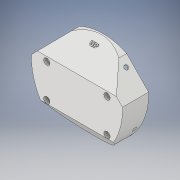
# Autodesk Inventor part: DGB Cover 2
Saved by Autodesk Inventor 2018 (Build 220112000, 112)
## iProperties
Created: 2019-02-18
Part Number: DGB Cover 2
Material: ABS Plastic
Document SubType Name: Modeling
Designer: Joe
Density: 1.06 g/cm^3
Appearance: Smooth - White
Author: Joe
Autodesk Inventor part; units mm, degrees
(part 1 of 16)
ref_plane "YZ Plane" through (0, 0, 0) normal (1, 0, 0) x (0, 1, 0)
ref_plane "Work Plane1" through (0, 0, 0) normal (0, 0, 1) x (1, 0, 0)
sketch "Sketch1" plane through (0, 0, 0) normal (0, 0, 1) x (1, 0, 0)
  arc A0 (-69.2264, 99.4238) -> (-77.754, 69.3573) centre (-45.7832, 76.5321) ccw
  line L0 (-61.6428, -2.4333) -> (-77.754, 69.3573)
  arc A1 (-61.6428, -2.4333) -> (-56.4257, -9.5833) centre (-50.8, 0) ccw
  line L1 (-56.4257, -9.5833) -> (-18.6452, -31.7617)
  arc A2 (-18.6452, -31.7617) -> (18.6452, -31.7617) centre (0, 0) ccw
  line L2 (56.4257, -9.5833) -> (18.6452, -31.7617)
  arc A3 (56.4257, -9.5833) -> (61.6428, -2.4333) centre (50.8, 0) ccw
  line L3 (77.754, 69.3573) -> (61.6428, -2.4333)
  arc A4 (77.754, 69.3573) -> (69.2264, 99.4238) centre (45.7832, 76.5321) ccw
  line L4 (69.2264, 99.4238) -> (23.4432, 146.3102)
  arc A5 (23.4432, 146.3102) -> (-23.4432, 146.3102) centre (0, 123.4186) ccw
  line L5 (-23.4432, 146.3102) -> (-69.2264, 99.4238)
  circle A6 centre (45.7832, 76.5321) radius 9.5631
  circle A7 centre (0, 123.4186) radius 9.5631
  circle A8 centre (63.5, 38.1) radius 2.4892
  circle A9 centre (0, 0) radius 14.2951
  circle A10 centre (0, 41.9862) radius 14.2951
  circle A11 centre (-63.5, 38.1) radius 2.4892
  circle A12 centre (50.8, 0) radius 2.4892
  circle A13 centre (-45.7832, 76.5321) radius 9.5631
  circle A14 centre (-50.8, 0) radius 2.4892
  arc A15 (60.8674, 81.4802) -> (51.089, 91.4942) centre (45.7832, 76.5321) ccw
  arc A16 (48.9582, 94.5106) -> (51.089, 91.4942) centre (52.1586, 94.5106) ccw
  line L6 (48.9582, 94.5106) -> (48.9582, 95.9294)
  arc A17 (49.8285, 98.1233) -> (48.9582, 95.9294) centre (52.1586, 95.9294) ccw
  arc A18 (49.8285, 98.1233) -> (51.2978, 101.2528) centre (45.7832, 101.9321) ccw
  arc A19 (56.764, 103.0974) -> (51.2978, 101.2528) centre (54.4742, 100.8615) ccw
  line L7 (56.764, 103.0974) -> (64.6832, 94.9874)
  arc A20 (71.3491, 83.1797) -> (64.6832, 94.9874) centre (45.7832, 76.5321) ccw
  arc A21 (68.1755, 79.1748) -> (71.3491, 83.1797) centre (68.2517, 82.3743) ccw
  line L8 (63.8322, 79.2782) -> (68.1755, 79.1748)
  arc A22 (60.8674, 81.4802) -> (63.8322, 79.2782) centre (63.9084, 82.4777) ccw
  arc A23 (42.8406, 46.4191) -> (46.4544, 45.6166) centre (45.7832, 51.1321) ccw
  arc A24 (48.7374, 45.0177) -> (46.4544, 45.6166) centre (46.841, 42.4396) ccw
  line L9 (56.7832, 39.0993) -> (48.7374, 45.0177)
  arc A25 (58.0348, 37.0983) -> (56.7832, 39.0993) centre (54.8868, 36.5212) ccw
  arc A26 (58.0348, 37.0983) -> (60.7938, 33.2473) centre (63.5, 38.1) ccw
  arc A27 (62.3577, 29.7514) -> (60.7938, 33.2473) centre (59.235, 30.4522) ccw
  line L10 (62.3577, 29.7514) -> (58.5623, 12.8393)
  arc A28 (54.4022, 10.5125) -> (58.5623, 12.8393) centre (55.4396, 13.5401) ccw
  arc A29 (54.4022, 10.5125) -> (49.4734, 11.033) centre (50.8, 0) ccw
  arc A30 (46.4166, 12.4531) -> (49.4734, 11.033) centre (49.0913, 14.2105) ccw
  line L11 (46.4166, 12.4531) -> (28.3641, 39.9279)
  arc A31 (30.4118, 44.8237) -> (28.3641, 39.9279) centre (31.0388, 41.6853) ccw
  line L12 (40.5187, 46.8427) -> (30.4118, 44.8237)
  arc A32 (42.8406, 46.4191) -> (40.5187, 46.8427) centre (41.1457, 43.7044) ccw
  arc A33 (30.699, 71.5841) -> (40.4775, 61.57) centre (45.7832, 76.5321) ccw
  arc A34 (42.6082, 58.5537) -> (40.4775, 61.57) centre (39.4078, 58.5537) ccw
  line L13 (42.6082, 58.5537) -> (42.6082, 57.1349)
  arc A35 (41.7379, 54.941) -> (42.6082, 57.1349) centre (39.4078, 57.1349) ccw
  arc A36 (41.7379, 54.941) -> (41.2557, 54.3529) centre (45.7832, 51.1321) ccw
  arc A37 (39.2748, 53.0697) -> (41.2557, 54.3529) centre (38.6478, 56.2081) ccw
  line L14 (39.2748, 53.0697) -> (20.2825, 49.2757)
  arc A38 (16.8284, 50.9142) -> (20.2825, 49.2757) centre (19.6555, 52.4141) ccw
  arc A39 (16.8284, 50.9142) -> (11.4097, 57.2414) centre (0, 41.9862) ccw
  arc A40 (11.4097, 62.3672) -> (11.4097, 57.2414) centre (13.3265, 59.8043) ccw
  arc A41 (11.4097, 62.3672) -> (18.1161, 71.7311) centre (0, 77.6224) ccw
  arc A42 (21.2358, 73.9408) -> (18.1161, 71.7311) centre (21.1597, 70.7413) ccw
  line L15 (21.2358, 73.9408) -> (27.7343, 73.7861)
  arc A43 (30.699, 71.5841) -> (27.7343, 73.7861) centre (27.6581, 70.5866) ccw
  arc A44 (4.0453, -22.2239) -> (5.3857, -19.781) centre (0, -18.415) ccw
  arc A45 (7.267, -17.6095) -> (5.3857, -19.781) centre (8.4879, -20.5678) ccw
  arc A46 (7.267, -17.6095) -> (17.7154, -7.0048) centre (0, 0) ccw
  arc A47 (21.8322, -5.1914) -> (17.7154, -7.0048) centre (20.6916, -8.1816) ccw
  arc A48 (21.8322, -5.1914) -> (27.6214, -4.0453) centre (23.8125, 0) ccw
  arc A49 (29.8153, -3.175) -> (27.6214, -4.0453) centre (29.8153, -6.3754) ccw
  line L16 (29.8153, -3.175) -> (37.9854, -3.175)
  arc A50 (40.8508, -4.9498) -> (37.9854, -3.175) centre (37.9854, -6.3754) ccw
  arc A51 (40.8508, -4.9498) -> (41.888, -6.638) centre (50.8, 0) ccw
  arc A52 (40.9415, -11.3097) -> (41.888, -6.638) centre (39.3213, -8.5498) ccw
  line L17 (40.9415, -11.3097) -> (15.4305, -26.2855)
  arc A53 (7.1234, -29.6359) -> (15.4305, -26.2855) centre (0, 0) ccw
  arc A54 (3.175, -26.5242) -> (7.1234, -29.6359) centre (6.3754, -26.5242) ccw
  line L18 (3.175, -24.4178) -> (3.175, -26.5242)
  arc A55 (4.0453, -22.2239) -> (3.175, -24.4178) centre (6.3754, -24.4178) ccw
  arc A56 (-27.6214, -4.0453) -> (-21.8322, -5.1914) centre (-23.8125, 0) ccw
  arc A57 (-17.7154, -7.0048) -> (-21.8322, -5.1914) centre (-20.6916, -8.1816) ccw
  arc A58 (-17.7154, -7.0048) -> (-7.267, -17.6095) centre (0, 0) ccw
  arc A59 (-5.3857, -19.781) -> (-7.267, -17.6095) centre (-8.4879, -20.5678) ccw
  arc A60 (-5.3857, -19.781) -> (-4.0453, -22.2239) centre (0, -18.415) ccw
  arc A61 (-3.175, -24.4178) -> (-4.0453, -22.2239) centre (-6.3754, -24.4178) ccw
  line L19 (-3.175, -24.4178) -> (-3.175, -26.5242)
  arc A62 (-7.1234, -29.6359) -> (-3.175, -26.5242) centre (-6.3754, -26.5242) ccw
  arc A63 (-15.4305, -26.2855) -> (-7.1234, -29.6359) centre (0, 0) ccw
  line L20 (-40.9415, -11.3097) -> (-15.4305, -26.2855)
  arc A64 (-41.888, -6.638) -> (-40.9415, -11.3097) centre (-39.3213, -8.5498) ccw
  arc A65 (-41.888, -6.638) -> (-40.8508, -4.9498) centre (-50.8, 0) ccw
  arc A66 (-37.9854, -3.175) -> (-40.8508, -4.9498) centre (-37.9854, -6.3754) ccw
  line L21 (-29.8153, -3.175) -> (-37.9854, -3.175)
  arc A67 (-27.6214, -4.0453) -> (-29.8153, -3.175) centre (-29.8153, -6.3754) ccw
  line L22 (-63.681, 72.93) -> (-68.1024, 72.8247)
  arc A68 (-60.6148, 70.8717) -> (-63.681, 72.93) centre (-63.6048, 69.7305) ccw
  arc A69 (-60.6148, 70.8717) -> (-51.089, 61.57) centre (-45.7832, 76.5321) ccw
  arc A70 (-48.9582, 58.5537) -> (-51.089, 61.57) centre (-52.1586, 58.5537) ccw
  line L23 (-48.9582, 58.5537) -> (-48.9582, 57.1349)
  arc A71 (-49.8285, 54.941) -> (-48.9582, 57.1349) centre (-52.1586, 57.1349) ccw
  arc A72 (-49.8285, 54.941) -> (-51.2484, 52.1339) centre (-45.7832, 51.1321) ccw
  arc A73 (-52.5, 50.1329) -> (-51.2484, 52.1339) centre (-54.3964, 52.7109) ccw
  line L24 (-60.5458, 44.2145) -> (-52.5, 50.1329)
  arc A74 (-62.8288, 43.6156) -> (-60.5458, 44.2145) centre (-62.4422, 46.7925) ccw
  arc A75 (-62.8288, 43.6156) -> (-63.1269, 43.6437) centre (-63.5, 38.1) ccw
  arc A76 (-66.0348, 46.1361) -> (-63.1269, 43.6437) centre (-62.9121, 46.8369) ccw
  line L25 (-71.1489, 68.9245) -> (-66.0348, 46.1361)
  arc A77 (-68.1024, 72.8247) -> (-71.1489, 68.9245) centre (-68.0262, 69.6253) ccw
  line L26 (-42.6082, 58.5537) -> (-42.6082, 57.1349)
  arc A78 (-40.4775, 61.57) -> (-42.6082, 58.5537) centre (-39.4078, 58.5537) ccw
  arc A79 (-40.4775, 61.57) -> (-30.699, 71.5841) centre (-45.7832, 76.5321) ccw
  arc A80 (-27.7343, 73.7861) -> (-30.699, 71.5841) centre (-27.6581, 70.5866) ccw
  line L27 (-21.2358, 73.9408) -> (-27.7343, 73.7861)
  arc A81 (-18.1161, 71.7311) -> (-21.2358, 73.9408) centre (-21.1597, 70.7413) ccw
  arc A82 (-18.1161, 71.7311) -> (-11.4097, 62.3672) centre (0, 77.6224) ccw
  arc A83 (-11.4097, 57.2414) -> (-11.4097, 62.3672) centre (-13.3265, 59.8043) ccw
  arc A84 (-11.4097, 57.2414) -> (-16.8284, 50.9142) centre (0, 41.9862) ccw
  arc A85 (-20.2825, 49.2757) -> (-16.8284, 50.9142) centre (-19.6555, 52.4141) ccw
  line L28 (-39.2748, 53.0697) -> (-20.2825, 49.2757)
  arc A86 (-41.2557, 54.3529) -> (-39.2748, 53.0697) centre (-38.6478, 56.2081) ccw
  arc A87 (-41.2557, 54.3529) -> (-41.7379, 54.941) centre (-45.7832, 51.1321) ccw
  arc A88 (-42.6082, 57.1349) -> (-41.7379, 54.941) centre (-39.4078, 57.1349) ccw
  arc A89 (-9.0745, 16.7498) -> (-11.6167, 15.0982) centre (0, 0) ccw
  arc A90 (-14.438, 14.5547) -> (-11.6167, 15.0982) centre (-13.5683, 17.6346) ccw
  arc A91 (-14.438, 14.5547) -> (-21.4952, 8.8934) centre (-15.9479, 9.2075) ccw
  arc A92 (-24.3696, 5.5282) -> (-21.4952, 8.8934) centre (-24.6905, 8.7125) ccw
  arc A93 (-24.3696, 5.5282) -> (-27.6214, 4.0453) centre (-23.8125, 0) ccw
  arc A94 (-29.8153, 3.175) -> (-27.6214, 4.0453) centre (-29.8153, 6.3754) ccw
  line L29 (-29.8153, 3.175) -> (-37.9854, 3.175)
  arc A95 (-40.8508, 4.9498) -> (-37.9854, 3.175) centre (-37.9854, 6.3754) ccw
  arc A96 (-40.8508, 4.9498) -> (-41.1998, 5.5968) centre (-50.8, 0) ccw
  arc A97 (-41.1097, 8.9661) -> (-41.1998, 5.5968) centre (-38.435, 7.2087) ccw
  line L30 (-41.1097, 8.9661) -> (-23.466, 35.8187)
  arc A98 (-17.8007, 35.2012) -> (-23.466, 35.8187) centre (-20.7913, 34.0613) ccw
  arc A99 (-17.8007, 35.2012) -> (-9.0745, 25.2364) centre (0, 41.9862) ccw
  arc A100 (-9.0745, 16.7498) -> (-9.0745, 25.2364) centre (-11.3734, 20.9931) ccw
  arc A101 (-60.7938, 33.2473) -> (-58.0348, 37.0983) centre (-63.5, 38.1) ccw
  arc A102 (-56.7832, 39.0993) -> (-58.0348, 37.0983) centre (-54.8868, 36.5212) ccw
  line L31 (-56.7832, 39.0993) -> (-48.7374, 45.0177)
  arc A103 (-46.4544, 45.6166) -> (-48.7374, 45.0177) centre (-46.841, 42.4396) ccw
  arc A104 (-46.4544, 45.6166) -> (-42.8406, 46.4191) centre (-45.7832, 51.1321) ccw
  arc A105 (-40.5187, 46.8427) -> (-42.8406, 46.4191) centre (-41.1457, 43.7044) ccw
  line L32 (-40.5187, 46.8427) -> (-30.4118, 44.8237)
  arc A106 (-28.3641, 39.9279) -> (-30.4118, 44.8237) centre (-31.0388, 41.6853) ccw
  line L33 (-46.4166, 12.4531) -> (-28.3641, 39.9279)
  arc A107 (-49.4734, 11.033) -> (-46.4166, 12.4531) centre (-49.0913, 14.2105) ccw
  arc A108 (-49.4734, 11.033) -> (-54.4022, 10.5125) centre (-50.8, 0) ccw
  arc A109 (-58.5623, 12.8393) -> (-54.4022, 10.5125) centre (-55.4396, 13.5401) ccw
  line L34 (-62.3577, 29.7514) -> (-58.5623, 12.8393)
  arc A110 (-60.7938, 33.2473) -> (-62.3577, 29.7514) centre (-59.235, 30.4522) ccw
  arc A111 (-5.4584, 95.8737) -> (-18.376, 82.6447) centre (0, 77.6224) ccw
  arc A112 (-21.387, 80.289) -> (-18.376, 82.6447) centre (-21.4632, 83.4885) ccw
  line L35 (-21.387, 80.289) -> (-27.8854, 80.1343)
  arc A113 (-30.9517, 82.1926) -> (-27.8854, 80.1343) centre (-27.9616, 83.3337) ccw
  arc A114 (-30.9517, 82.1926) -> (-40.4775, 91.4942) centre (-45.7832, 76.5321) ccw
  arc A115 (-42.6082, 94.5106) -> (-40.4775, 91.4942) centre (-39.4078, 94.5106) ccw
  line L36 (-42.6082, 94.5106) -> (-42.6082, 95.9294)
  arc A116 (-41.7379, 98.1233) -> (-42.6082, 95.9294) centre (-39.4078, 95.9294) ccw
  arc A117 (-41.7379, 98.1233) -> (-41.6751, 105.6731) centre (-45.7832, 101.9321) ccw
  arc A118 (-42.5017, 108.0467) -> (-41.6751, 105.6731) centre (-39.3088, 107.8279) ccw
  line L37 (-42.5017, 108.0467) -> (-42.3115, 110.8224)
  arc A119 (-34.2504, 119.5866) -> (-42.3115, 110.8224) centre (-32.8088, 110.1713) ccw
  line L38 (-34.2504, 119.5866) -> (-31.6435, 119.9858)
  arc A120 (-29.0542, 119.2331) -> (-31.6435, 119.9858) centre (-31.1591, 116.8223) ccw
  arc A121 (-29.0542, 119.2331) -> (-21.5911, 119.3733) centre (-25.4, 123.4186) ccw
  arc A122 (-19.3972, 120.2436) -> (-21.5911, 119.3733) centre (-19.3972, 117.0432) ccw
  line L39 (-17.9785, 120.2436) -> (-19.3972, 120.2436)
  arc A123 (-14.9621, 118.1128) -> (-17.9785, 120.2436) centre (-17.9785, 117.0432) ccw
  arc A124 (-14.9621, 118.1128) -> (-5.3058, 108.4565) centre (0, 123.4186) ccw
  arc A125 (-3.175, 105.4401) -> (-5.3058, 108.4565) centre (-6.3754, 105.4401) ccw
  line L40 (-3.175, 105.4401) -> (-3.175, 98.9399)
  arc A126 (-5.4584, 95.8737) -> (-3.175, 98.9399) centre (-6.3754, 98.9399) ccw
  line L41 (-48.9582, 94.5106) -> (-48.9582, 95.9294)
  arc A127 (-51.089, 91.4942) -> (-48.9582, 94.5106) centre (-52.1586, 94.5106) ccw
  arc A128 (-51.089, 91.4942) -> (-60.8674, 81.4802) centre (-45.7832, 76.5321) ccw
  arc A129 (-63.8322, 79.2782) -> (-60.8674, 81.4802) centre (-63.9084, 82.4777) ccw
  line L42 (-63.8322, 79.2782) -> (-68.1755, 79.1748)
  arc A130 (-71.3491, 83.1797) -> (-68.1755, 79.1748) centre (-68.2517, 82.3743) ccw
  arc A131 (-64.6832, 94.9874) -> (-71.3491, 83.1797) centre (-45.7832, 76.5321) ccw
  line L43 (-56.764, 103.0974) -> (-64.6832, 94.9874)
  arc A132 (-51.2978, 101.2528) -> (-56.764, 103.0974) centre (-54.4742, 100.8615) ccw
  arc A133 (-51.2978, 101.2528) -> (-49.8285, 98.1233) centre (-45.7832, 101.9321) ccw
  arc A134 (-48.9582, 95.9294) -> (-49.8285, 98.1233) centre (-52.1586, 95.9294) ccw
  arc A135 (-5.3058, 138.3807) -> (-14.9621, 128.7244) centre (0, 123.4186) ccw
  arc A136 (-17.9785, 126.5936) -> (-14.9621, 128.7244) centre (-17.9785, 129.794) ccw
  line L44 (-17.9785, 126.5936) -> (-19.3972, 126.5936)
  arc A137 (-21.5911, 127.4639) -> (-19.3972, 126.5936) centre (-19.3972, 129.794) ccw
  arc A138 (-21.5911, 127.4639) -> (-24.5156, 128.904) centre (-25.4, 123.4186) ccw
  arc A139 (-26.2961, 134.2995) -> (-24.5156, 128.904) centre (-24.0062, 132.0636) ccw
  line L45 (-18.9, 141.8739) -> (-26.2961, 134.2995)
  arc A140 (-7.2543, 148.819) -> (-18.9, 141.8739) centre (0, 123.4186) ccw
  arc A141 (-3.175, 145.7416) -> (-7.2543, 148.819) centre (-6.3754, 145.7416) ccw
  line L46 (-3.175, 145.7416) -> (-3.175, 141.3971)
  arc A142 (-5.3058, 138.3807) -> (-3.175, 141.3971) centre (-6.3754, 141.3971) ccw
  arc A143 (51.089, 61.57) -> (60.6148, 70.8717) centre (45.7832, 76.5321) ccw
  arc A144 (63.681, 72.93) -> (60.6148, 70.8717) centre (63.6048, 69.7305) ccw
  line L47 (63.681, 72.93) -> (68.1024, 72.8247)
  arc A145 (71.1489, 68.9245) -> (68.1024, 72.8247) centre (68.0262, 69.6253) ccw
  line L48 (71.1489, 68.9245) -> (66.0348, 46.1361)
  arc A146 (63.1269, 43.6437) -> (66.0348, 46.1361) centre (62.9121, 46.8369) ccw
  arc A147 (63.1269, 43.6437) -> (62.8288, 43.6156) centre (63.5, 38.1) ccw
  arc A148 (60.5458, 44.2145) -> (62.8288, 43.6156) centre (62.4422, 46.7925) ccw
  line L49 (60.5458, 44.2145) -> (52.5, 50.1329)
  arc A149 (51.2484, 52.1339) -> (52.5, 50.1329) centre (54.3964, 52.7109) ccw
  arc A150 (51.2484, 52.1339) -> (49.8285, 54.941) centre (45.7832, 51.1321) ccw
  arc A151 (48.9582, 57.1349) -> (49.8285, 54.941) centre (52.1586, 57.1349) ccw
  line L50 (48.9582, 58.5537) -> (48.9582, 57.1349)
  arc A152 (51.089, 61.57) -> (48.9582, 58.5537) centre (52.1586, 58.5537) ccw
  arc A153 (21.4952, 8.8934) -> (14.438, 14.5547) centre (15.9479, 9.2075) ccw
  arc A154 (11.6167, 15.0982) -> (14.438, 14.5547) centre (13.5683, 17.6346) ccw
  arc A155 (11.6167, 15.0982) -> (9.0745, 16.7498) centre (0, 0) ccw
  arc A156 (9.0745, 25.2364) -> (9.0745, 16.7498) centre (11.3734, 20.9931) ccw
  arc A157 (9.0745, 25.2364) -> (17.8007, 35.2012) centre (0, 41.9862) ccw
  arc A158 (23.466, 35.8187) -> (17.8007, 35.2012) centre (20.7913, 34.0613) ccw
  line L51 (41.1097, 8.9661) -> (23.466, 35.8187)
  arc A159 (41.1998, 5.5968) -> (41.1097, 8.9661) centre (38.435, 7.2087) ccw
  arc A160 (41.1998, 5.5968) -> (40.8508, 4.9498) centre (50.8, 0) ccw
  arc A161 (37.9854, 3.175) -> (40.8508, 4.9498) centre (37.9854, 6.3754) ccw
  line L52 (29.8153, 3.175) -> (37.9854, 3.175)
  arc A162 (27.6214, 4.0453) -> (29.8153, 3.175) centre (29.8153, 6.3754) ccw
  arc A163 (27.6214, 4.0453) -> (24.3696, 5.5282) centre (23.8125, 0) ccw
  arc A164 (21.4952, 8.8934) -> (24.3696, 5.5282) centre (24.6905, 8.7125) ccw
  arc A165 (40.4775, 91.4942) -> (30.9517, 82.1926) centre (45.7832, 76.5321) ccw
  arc A166 (27.8854, 80.1343) -> (30.9517, 82.1926) centre (27.9616, 83.3337) ccw
  line L53 (21.387, 80.289) -> (27.8854, 80.1343)
  arc A167 (18.376, 82.6447) -> (21.387, 80.289) centre (21.4632, 83.4885) ccw
  arc A168 (18.376, 82.6447) -> (5.4584, 95.8737) centre (0, 77.6224) ccw
  arc A169 (3.175, 98.9399) -> (5.4584, 95.8737) centre (6.3754, 98.9399) ccw
  line L54 (3.175, 105.4401) -> (3.175, 98.9399)
  arc A170 (5.3058, 108.4565) -> (3.175, 105.4401) centre (6.3754, 105.4401) ccw
  arc A171 (5.3058, 108.4565) -> (14.9621, 118.1128) centre (0, 123.4186) ccw
  arc A172 (17.9785, 120.2436) -> (14.9621, 118.1128) centre (17.9785, 117.0432) ccw
  line L55 (17.9785, 120.2436) -> (19.3972, 120.2436)
  arc A173 (21.5911, 119.3733) -> (19.3972, 120.2436) centre (19.3972, 117.0432) ccw
  arc A174 (21.5911, 119.3733) -> (29.0542, 119.2331) centre (25.4, 123.4186) ccw
  arc A175 (31.6435, 119.9858) -> (29.0542, 119.2331) centre (31.1591, 116.8223) ccw
  line L56 (34.2504, 119.5866) -> (31.6435, 119.9858)
  arc A176 (42.3115, 110.8224) -> (34.2504, 119.5866) centre (32.8088, 110.1713) ccw
  line L57 (42.5017, 108.0467) -> (42.3115, 110.8224)
  arc A177 (41.6751, 105.6731) -> (42.5017, 108.0467) centre (39.3088, 107.8279) ccw
  arc A178 (41.6751, 105.6731) -> (41.7379, 98.1233) centre (45.7832, 101.9321) ccw
  arc A179 (42.6082, 95.9294) -> (41.7379, 98.1233) centre (39.4078, 95.9294) ccw
  line L58 (42.6082, 94.5106) -> (42.6082, 95.9294)
  arc A180 (40.4775, 91.4942) -> (42.6082, 94.5106) centre (39.4078, 94.5106) ccw
  arc A181 (24.5156, 128.904) -> (21.5911, 127.4639) centre (25.4, 123.4186) ccw
  arc A182 (19.3972, 126.5936) -> (21.5911, 127.4639) centre (19.3972, 129.794) ccw
  line L59 (17.9785, 126.5936) -> (19.3972, 126.5936)
  arc A183 (14.9621, 128.7244) -> (17.9785, 126.5936) centre (17.9785, 129.794) ccw
  arc A184 (14.9621, 128.7244) -> (5.3058, 138.3807) centre (0, 123.4186) ccw
  arc A185 (3.175, 141.3971) -> (5.3058, 138.3807) centre (6.3754, 141.3971) ccw
  line L60 (3.175, 145.7416) -> (3.175, 141.3971)
  arc A186 (7.2543, 148.819) -> (3.175, 145.7416) centre (6.3754, 145.7416) ccw
  arc A187 (18.9, 141.8739) -> (7.2543, 148.819) centre (0, 123.4186) ccw
  line L61 (18.9, 141.8739) -> (26.2961, 134.2995)
  arc A188 (24.5156, 128.904) -> (26.2961, 134.2995) centre (24.0062, 132.0636) ccw
  circle A189 centre (-45.7832, 51.1321) radius 2.4892
  circle A190 centre (45.7832, 51.1321) radius 2.4892
  circle A191 centre (45.7832, 101.9321) radius 2.4892
  circle A192 centre (25.4, 123.4186) radius 2.4892
  circle A193 centre (-25.4, 123.4186) radius 2.4892
  circle A194 centre (-45.7832, 101.9321) radius 2.4892
  circle A195 centre (15.9479, 9.2075) radius 2.0193
  circle A196 centre (0, -18.415) radius 2.0193
  circle A197 centre (-15.9479, 9.2075) radius 2.0193
  circle A198 centre (23.8125, 0) radius 2.0193
  circle A199 centre (-23.8125, 0) radius 2.0193
  circle A200 centre (0, 77.6224) radius 14.2951
  arc A201 (34.312, 96.9978) -> (33.7262, 97.9989) centre (0.0435, 77.6158) ccw
  spline S0 degree 3 poles (32.0983, 100.4737) (32.0228, 100.362) (31.9457, 100.2513) (31.8668, 100.1419) (31.8241, 100.0828) (31.7809, 100.024) (31.7372, 99.9657) (31.6959, 99.9104) (31.654, 99.8555) (31.6117, 99.801) (31.5717, 99.7496) (31.5313, 99.6985) (31.4905, 99.6478) (31.452, 99.6001) (31.4132, 99.5527) (31.3739, 99.5057) (31.3371, 99.4617) (31.3, 99.418) (31.2624, 99.3746) (31.2274, 99.3342) (31.192, 99.2941) (31.1563, 99.2543) (31.1232, 99.2174) (31.0897, 99.1808) (31.056, 99.1445) (31.0248, 99.111) (30.9934, 99.0778) (30.9617, 99.0449) (30.9327, 99.0148) (30.9034, 98.9849) (30.8738, 98.9553) (30.847, 98.9285) (30.82, 98.9019) (30.7927, 98.8755) (30.7682, 98.8519) (30.7435, 98.8284) (30.7186, 98.8052) (30.6857, 98.7746) (30.6523, 98.7444) (30.6187, 98.7145) (30.6112, 98.7078) (30.6037, 98.7011) (30.5962, 98.6943) (30.5889, 98.6877) (30.5817, 98.6811) (30.5745, 98.6743) (30.5675, 98.6677) (30.5605, 98.6611) (30.5536, 98.6543) (30.5469, 98.6478) (30.5402, 98.6411) (30.5336, 98.6344) (30.527, 98.6278) (30.5206, 98.6212) (30.5142, 98.6144) (30.5079, 98.6078) (30.5017, 98.6012) (30.4956, 98.5944) (30.4895, 98.5877) (30.4836, 98.581) (30.4777, 98.5742) (30.4718, 98.5675) (30.466, 98.5607) (30.4604, 98.5538) (30.4547, 98.5469) (30.4492, 98.54) (30.4437, 98.533) (30.4382, 98.5259) (30.4329, 98.5188) (30.4276, 98.5116) (30.4223, 98.5044) (30.4171, 98.497) (30.4121, 98.4896) (30.4069, 98.4821) (30.4019, 98.4744) (30.397, 98.4667) (30.392, 98.4587) (30.3872, 98.4506) (30.3825, 98.4424) (30.3776, 98.4339) (30.373, 98.4253) (30.3685, 98.4166) (30.3638, 98.4074) (30.3593, 98.3981) (30.3551, 98.3886) (30.3506, 98.3785) (30.3464, 98.3683) (30.3425, 98.3579) (30.3382, 98.3467) (30.3344, 98.3352) (30.3309, 98.3237) (30.3272, 98.311) (30.3239, 98.2981) (30.3211, 98.2851) (30.3181, 98.2706) (30.3157, 98.256) (30.3141, 98.2413) (30.3122, 98.2247) (30.3112, 98.2081) (30.3112, 98.1914) (30.3112, 98.1727) (30.3124, 98.154) (30.3148, 98.1354) (30.3175, 98.1148) (30.3217, 98.0944) (30.3273, 98.0743) (30.3334, 98.0526) (30.3412, 98.0313) (30.3508, 98.0109) (30.36, 97.9914) (30.3709, 97.9728) (30.3821, 97.9544) (30.4375, 97.8633) (30.5003, 97.7772) (30.5588, 97.6882) (30.6174, 97.5993) (30.6715, 97.5075) (30.7333, 97.4205) (30.7457, 97.403) (30.7585, 97.3856) (30.7728, 97.3694) (30.7876, 97.3525) (30.8041, 97.3369) (30.8217, 97.3227) (30.8378, 97.3096) (30.8549, 97.2977) (30.8728, 97.2871) (30.8889, 97.2775) (30.9056, 97.269) (30.9228, 97.2616) (30.9381, 97.255) (30.9538, 97.2493) (30.9698, 97.2445) (30.9839, 97.2401) (30.9983, 97.2365) (31.0128, 97.2336) (31.0258, 97.231) (31.039, 97.2289) (31.0521, 97.2273) (31.0641, 97.2259) (31.0761, 97.2249) (31.0881, 97.2243) (31.0992, 97.2238) (31.1102, 97.2236) (31.1213, 97.2238) (31.1316, 97.2239) (31.142, 97.2243) (31.1523, 97.225) (31.1621, 97.2257) (31.1718, 97.2265) (31.1816, 97.2276) (31.1909, 97.2287) (31.2003, 97.23) (31.2096, 97.2314) (31.2186, 97.2328) (31.2276, 97.2344) (31.2366, 97.2361) (31.2454, 97.2378) (31.2542, 97.2397) (31.263, 97.2417) (31.2717, 97.2436) (31.2803, 97.2458) (31.2889, 97.248) (31.2975, 97.2502) (31.3061, 97.2526) (31.3146, 97.2551) (31.3232, 97.2575) (31.3317, 97.2601) (31.3402, 97.2628) (31.3488, 97.2656) (31.3574, 97.2684) (31.3659, 97.2713) (31.3745, 97.2743) (31.3831, 97.2773) (31.3917, 97.2805) (31.4004, 97.2837) (31.409, 97.287) (31.4177, 97.2903) (31.4264, 97.2938) (31.4352, 97.2973) (31.4439, 97.3009) (31.4528, 97.3046) (31.4617, 97.3083) (31.4705, 97.3121) (31.4796, 97.3161) (31.4886, 97.32) (31.4975, 97.3241) (31.5067, 97.3283) (31.5158, 97.3326) (31.5249, 97.3368) (31.5657, 97.3558) (31.6066, 97.3745) (31.6478, 97.3926) (31.679, 97.4063) (31.7103, 97.4197) (31.7417, 97.4328) (31.7767, 97.4474) (31.8119, 97.4617) (31.8471, 97.4757) (31.886, 97.4911) (31.925, 97.5062) (31.9641, 97.5209) (32.0069, 97.537) (32.0498, 97.5527) (32.0929, 97.5681) (32.1396, 97.5847) (32.1865, 97.6009) (32.2335, 97.6167) (32.2842, 97.6338) (32.335, 97.6504) (32.386, 97.6665) (32.4407, 97.6838) (32.4955, 97.7006) (32.5505, 97.717) (32.6092, 97.7344) (32.6681, 97.7513) (32.7271, 97.7677) (32.7899, 97.7852) (32.8528, 97.802) (32.9158, 97.8184) (32.9827, 97.8357) (33.0496, 97.8524) (33.1168, 97.8685) (33.1877, 97.8855) (33.2587, 97.9018) (33.3299, 97.9176) (33.4616, 97.9467) (33.5937, 97.9738) (33.7262, 97.9989) knots 0 0 0 0 0.057795 0.057795 0.057795 0.089038 0.089038 0.089038 0.118617 0.118617 0.118617 0.14653 0.14653 0.14653 0.172778 0.172778 0.172778 0.19736 0.19736 0.19736 0.220277 0.220277 0.220277 0.241529 0.241529 0.241529 0.261115 0.261115 0.261115 0.279036 0.279036 0.279036 0.295292 0.295292 0.295292 0.309882 0.309882 0.309882 0.329164 0.329164 0.329164 0.333477 0.333477 0.333477 0.337694 0.337694 0.337694 0.34182 0.34182 0.34182 0.345864 0.345864 0.345864 0.349834 0.349834 0.349834 0.353742 0.353742 0.353742 0.3576 0.3576 0.3576 0.361424 0.361424 0.361424 0.365232 0.365232 0.365232 0.369048 0.369048 0.369048 0.372899 0.372899 0.372899 0.376819 0.376819 0.376819 0.380853 0.380853 0.380853 0.385052 0.385052 0.385052 0.389482 0.389482 0.389482 0.394225 0.394225 0.394225 0.399381 0.399381 0.399381 0.405067 0.405067 0.405067 0.411413 0.411413 0.411413 0.418548 0.418548 0.418548 0.426565 0.426565 0.426565 0.435472 0.435472 0.435472 0.445133 0.445133 0.445133 0.45436 0.45436 0.45436 0.5 0.5 0.5 0.54564 0.54564 0.54564 0.554867 0.554867 0.554867 0.564528 0.564528 0.564528 0.573435 0.573435 0.573435 0.581452 0.581452 0.581452 0.588587 0.588587 0.588587 0.594933 0.594933 0.594933 0.600619 0.600619 0.600619 0.605775 0.605775 0.605775 0.610518 0.610518 0.610518 0.614948 0.614948 0.614948 0.619147 0.619147 0.619147 0.623181 0.623181 0.623181 0.627101 0.627101 0.627101 0.630952 0.630952 0.630952 0.634768 0.634768 0.634768 0.638576 0.638576 0.638576 0.6424 0.6424 0.6424 0.646258 0.646258 0.646258 0.650166 0.650166 0.650166 0.654136 0.654136 0.654136 0.65818 0.65818 0.65818 0.662306 0.662306 0.662306 0.666523 0.666523 0.666523 0.670836 0.670836 0.670836 0.690118 0.690118 0.690118 0.704708 0.704708 0.704708 0.720964 0.720964 0.720964 0.738885 0.738885 0.738885 0.758471 0.758471 0.758471 0.779723 0.779723 0.779723 0.80264 0.80264 0.80264 0.827222 0.827222 0.827222 0.85347 0.85347 0.85347 0.881383 0.881383 0.881383 0.910962 0.910962 0.910962 0.942205 0.942205 0.942205 1 1 1 1
  arc A202 (32.0983, 100.4737) -> (31.4111, 101.408) centre (0.0435, 77.6158) ccw
  spline S1 degree 3 poles (29.5334, 103.6991) (29.47, 103.5801) (29.4048, 103.462) (29.3378, 103.345) (29.3016, 103.2817) (29.2648, 103.2188) (29.2274, 103.1561) (29.1921, 103.0969) (29.1562, 103.0379) (29.1198, 102.9793) (29.0854, 102.9239) (29.0506, 102.8689) (29.0152, 102.8142) (28.982, 102.7627) (28.9483, 102.7116) (28.9142, 102.6607) (28.8822, 102.6131) (28.8498, 102.5657) (28.817, 102.5187) (28.7864, 102.4748) (28.7554, 102.4312) (28.724, 102.3879) (28.695, 102.3478) (28.6655, 102.3079) (28.6357, 102.2682) (28.6083, 102.2317) (28.5805, 102.1954) (28.5524, 102.1593) (28.5266, 102.1264) (28.5007, 102.0936) (28.4743, 102.0611) (28.4505, 102.0316) (28.4264, 102.0023) (28.402, 101.9733) (28.3801, 101.9472) (28.358, 101.9212) (28.3357, 101.8956) (28.3061, 101.8616) (28.2761, 101.8281) (28.2458, 101.7949) (28.239, 101.7874) (28.2322, 101.78) (28.2255, 101.7725) (28.219, 101.7652) (28.2125, 101.7578) (28.206, 101.7503) (28.1998, 101.743) (28.1935, 101.7357) (28.1874, 101.7283) (28.1813, 101.721) (28.1754, 101.7137) (28.1695, 101.7063) (28.1637, 101.6991) (28.158, 101.6918) (28.1523, 101.6845) (28.1468, 101.6772) (28.1413, 101.6699) (28.1359, 101.6626) (28.1306, 101.6553) (28.1253, 101.648) (28.1202, 101.6406) (28.1151, 101.6333) (28.1101, 101.6259) (28.1051, 101.6185) (28.1002, 101.6111) (28.0954, 101.6036) (28.0907, 101.5961) (28.086, 101.5885) (28.0814, 101.5809) (28.077, 101.5732) (28.0724, 101.5654) (28.068, 101.5576) (28.0638, 101.5496) (28.0595, 101.5416) (28.0553, 101.5335) (28.0512, 101.5252) (28.0471, 101.5168) (28.0431, 101.5083) (28.0393, 101.4996) (28.0354, 101.4907) (28.0316, 101.4816) (28.0281, 101.4725) (28.0244, 101.4628) (28.0209, 101.4531) (28.0177, 101.4433) (28.0142, 101.4327) (28.0111, 101.4221) (28.0083, 101.4114) (28.0053, 101.3998) (28.0027, 101.388) (28.0005, 101.3762) (27.998, 101.3631) (27.9961, 101.35) (27.9947, 101.3368) (27.9932, 101.322) (27.9924, 101.3072) (27.9923, 101.2924) (27.9922, 101.2758) (27.9929, 101.2591) (27.9947, 101.2425) (27.9966, 101.2239) (27.9998, 101.2054) (28.0041, 101.1872) (28.0089, 101.167) (28.0152, 101.1471) (28.0229, 101.1278) (28.0312, 101.1068) (28.0412, 101.0864) (28.0529, 101.0671) (28.0641, 101.0488) (28.0769, 101.0314) (28.0899, 101.0142) (28.1545, 100.9294) (28.226, 100.8503) (28.2935, 100.768) (28.361, 100.6856) (28.4245, 100.6) (28.495, 100.52) (28.5092, 100.5038) (28.5238, 100.4879) (28.5396, 100.4733) (28.5562, 100.458) (28.5742, 100.4442) (28.5931, 100.4319) (28.6106, 100.4206) (28.6288, 100.4105) (28.6477, 100.4018) (28.6647, 100.394) (28.6823, 100.3873) (28.7001, 100.3818) (28.716, 100.3768) (28.7322, 100.3728) (28.7486, 100.3696) (28.7631, 100.3668) (28.7778, 100.3647) (28.7926, 100.3633) (28.8058, 100.362) (28.819, 100.3613) (28.8323, 100.3612) (28.8443, 100.361) (28.8564, 100.3613) (28.8684, 100.362) (28.8794, 100.3626) (28.8905, 100.3636) (28.9015, 100.3649) (28.9117, 100.3661) (28.922, 100.3676) (28.9322, 100.3693) (28.9418, 100.371) (28.9514, 100.3729) (28.961, 100.375) (28.9702, 100.377) (28.9793, 100.3793) (28.9884, 100.3817) (28.9973, 100.384) (29.0061, 100.3865) (29.0148, 100.3892) (29.0234, 100.3918) (29.032, 100.3946) (29.0405, 100.3975) (29.0489, 100.4004) (29.0573, 100.4034) (29.0656, 100.4065) (29.074, 100.4096) (29.0822, 100.4129) (29.0905, 100.4162) (29.0987, 100.4196) (29.1069, 100.423) (29.1151, 100.4266) (29.1234, 100.4302) (29.1316, 100.4339) (29.1397, 100.4377) (29.148, 100.4416) (29.1562, 100.4455) (29.1644, 100.4495) (29.1727, 100.4536) (29.181, 100.4578) (29.1892, 100.462) (29.1976, 100.4664) (29.206, 100.4708) (29.2143, 100.4753) (29.2227, 100.4799) (29.2311, 100.4845) (29.2395, 100.4893) (29.2481, 100.4941) (29.2566, 100.499) (29.2651, 100.504) (29.2738, 100.5091) (29.2824, 100.5143) (29.291, 100.5195) (29.3296, 100.5427) (29.3684, 100.5655) (29.4074, 100.5878) (29.437, 100.6047) (29.4667, 100.6213) (29.4966, 100.6376) (29.5299, 100.6558) (29.5634, 100.6737) (29.597, 100.6913) (29.634, 100.7107) (29.6712, 100.7298) (29.7086, 100.7485) (29.7495, 100.769) (29.7905, 100.7891) (29.8317, 100.8088) (29.8765, 100.8303) (29.9214, 100.8513) (29.9665, 100.8719) (30.0151, 100.8942) (30.0639, 100.916) (30.113, 100.9374) (30.1655, 100.9603) (30.2183, 100.9828) (30.2713, 101.0048) (30.3279, 101.0283) (30.3846, 101.0512) (30.4416, 101.0737) (30.5022, 101.0976) (30.563, 101.121) (30.624, 101.1438) (30.6887, 101.168) (30.7535, 101.1916) (30.8186, 101.2146) (30.8873, 101.2389) (30.9563, 101.2627) (31.0254, 101.2858) (31.1533, 101.3285) (31.2819, 101.3692) (31.4111, 101.408) knots 0 0 0 0 0.057795 0.057795 0.057795 0.089038 0.089038 0.089038 0.118617 0.118617 0.118617 0.14653 0.14653 0.14653 0.172778 0.172778 0.172778 0.19736 0.19736 0.19736 0.220277 0.220277 0.220277 0.241529 0.241529 0.241529 0.261115 0.261115 0.261115 0.279036 0.279036 0.279036 0.295292 0.295292 0.295292 0.309882 0.309882 0.309882 0.329164 0.329164 0.329164 0.333477 0.333477 0.333477 0.337694 0.337694 0.337694 0.34182 0.34182 0.34182 0.345864 0.345864 0.345864 0.349834 0.349834 0.349834 0.353742 0.353742 0.353742 0.3576 0.3576 0.3576 0.361424 0.361424 0.361424 0.365232 0.365232 0.365232 0.369048 0.369048 0.369048 0.372899 0.372899 0.372899 0.376819 0.376819 0.376819 0.380853 0.380853 0.380853 0.385052 0.385052 0.385052 0.389482 0.389482 0.389482 0.394225 0.394225 0.394225 0.399381 0.399381 0.399381 0.405067 0.405067 0.405067 0.411413 0.411413 0.411413 0.418548 0.418548 0.418548 0.426565 0.426565 0.426565 0.435472 0.435472 0.435472 0.445133 0.445133 0.445133 0.45436 0.45436 0.45436 0.5 0.5 0.5 0.54564 0.54564 0.54564 0.554867 0.554867 0.554867 0.564528 0.564528 0.564528 0.573435 0.573435 0.573435 0.581452 0.581452 0.581452 0.588587 0.588587 0.588587 0.594933 0.594933 0.594933 0.600619 0.600619 0.600619 0.605775 0.605775 0.605775 0.610518 0.610518 0.610518 0.614948 0.614948 0.614948 0.619147 0.619147 0.619147 0.623181 0.623181 0.623181 0.627101 0.627101 0.627101 0.630952 0.630952 0.630952 0.634768 0.634768 0.634768 0.638576 0.638576 0.638576 0.6424 0.6424 0.6424 0.646258 0.646258 0.646258 0.650166 0.650166 0.650166 0.654136 0.654136 0.654136 0.65818 0.65818 0.65818 0.662306 0.662306 0.662306 0.666523 0.666523 0.666523 0.670836 0.670836 0.670836 0.690118 0.690118 0.690118 0.704708 0.704708 0.704708 0.720964 0.720964 0.720964 0.738885 0.738885 0.738885 0.758471 0.758471 0.758471 0.779723 0.779723 0.779723 0.80264 0.80264 0.80264 0.827222 0.827222 0.827222 0.85347 0.85347 0.85347 0.881383 0.881383 0.881383 0.910962 0.910962 0.910962 0.942205 0.942205 0.942205 1 1 1 1
  arc A203 (29.5334, 103.6991) -> (28.7523, 104.5565) centre (0.0435, 77.6158) ccw
  spline S2 degree 3 poles (26.6454, 106.6388) (26.5948, 106.5138) (26.5423, 106.3895) (26.4879, 106.2661) (26.4585, 106.1994) (26.4285, 106.133) (26.3979, 106.0668) (26.3689, 106.0041) (26.3394, 105.9417) (26.3093, 105.8796) (26.2809, 105.821) (26.252, 105.7626) (26.2226, 105.7045) (26.1949, 105.6499) (26.1667, 105.5955) (26.1381, 105.5413) (26.1113, 105.4906) (26.084, 105.4401) (26.0563, 105.3899) (26.0304, 105.3431) (26.0042, 105.2965) (25.9775, 105.2502) (25.9528, 105.2072) (25.9277, 105.1644) (25.9022, 105.1219) (25.8787, 105.0827) (25.8549, 105.0437) (25.8307, 105.0049) (25.8086, 104.9694) (25.7861, 104.9341) (25.7634, 104.899) (25.7427, 104.8672) (25.7218, 104.8355) (25.7006, 104.8041) (25.6816, 104.7759) (25.6623, 104.7478) (25.6428, 104.7199) (25.6169, 104.6831) (25.5906, 104.6466) (25.5639, 104.6104) (25.5579, 104.6023) (25.552, 104.5942) (25.5461, 104.586) (25.5403, 104.578) (25.5346, 104.57) (25.529, 104.5619) (25.5235, 104.554) (25.5181, 104.546) (25.5128, 104.538) (25.5075, 104.5302) (25.5023, 104.5223) (25.4973, 104.5143) (25.4922, 104.5065) (25.4873, 104.4987) (25.4825, 104.4908) (25.4777, 104.483) (25.473, 104.4752) (25.4684, 104.4673) (25.4639, 104.4595) (25.4594, 104.4517) (25.4551, 104.4438) (25.4508, 104.436) (25.4466, 104.4282) (25.4424, 104.4202) (25.4383, 104.4124) (25.4343, 104.4044) (25.4305, 104.3964) (25.4266, 104.3884) (25.4228, 104.3804) (25.4192, 104.3722) (25.4155, 104.364) (25.4119, 104.3558) (25.4085, 104.3475) (25.4051, 104.339) (25.4017, 104.3305) (25.3986, 104.3219) (25.3953, 104.313) (25.3923, 104.3041) (25.3894, 104.2952) (25.3864, 104.2858) (25.3836, 104.2764) (25.3811, 104.267) (25.3784, 104.257) (25.3759, 104.2469) (25.3738, 104.2368) (25.3715, 104.226) (25.3695, 104.2151) (25.3678, 104.2042) (25.366, 104.1923) (25.3646, 104.1803) (25.3637, 104.1683) (25.3626, 104.1551) (25.3621, 104.1418) (25.3621, 104.1285) (25.3621, 104.1137) (25.3629, 104.0989) (25.3643, 104.0842) (25.3659, 104.0676) (25.3684, 104.0511) (25.3719, 104.0348) (25.3758, 104.0165) (25.3808, 103.9984) (25.387, 103.9808) (25.3939, 103.9611) (25.4023, 103.942) (25.4119, 103.9236) (25.4224, 103.9036) (25.4345, 103.8844) (25.4481, 103.8665) (25.4612, 103.8493) (25.4757, 103.8334) (25.4905, 103.8177) (25.5636, 103.7401) (25.643, 103.6689) (25.7187, 103.5941) (25.7944, 103.5193) (25.8665, 103.4407) (25.945, 103.3685) (25.9608, 103.3539) (25.977, 103.3396) (25.9942, 103.3267) (26.0123, 103.3133) (26.0317, 103.3015) (26.0518, 103.2912) (26.0703, 103.2818) (26.0895, 103.2736) (26.1092, 103.267) (26.127, 103.261) (26.1451, 103.2561) (26.1635, 103.2525) (26.1798, 103.2492) (26.1963, 103.2469) (26.2129, 103.2455) (26.2277, 103.2442) (26.2425, 103.2436) (26.2573, 103.2438) (26.2706, 103.2439) (26.2838, 103.2446) (26.2971, 103.2458) (26.309, 103.2469) (26.321, 103.2485) (26.3329, 103.2504) (26.3438, 103.2522) (26.3547, 103.2543) (26.3654, 103.2567) (26.3755, 103.259) (26.3856, 103.2616) (26.3955, 103.2644) (26.4049, 103.2671) (26.4143, 103.2699) (26.4236, 103.273) (26.4325, 103.276) (26.4414, 103.2792) (26.4502, 103.2825) (26.4587, 103.2858) (26.4672, 103.2892) (26.4757, 103.2928) (26.4839, 103.2963) (26.4921, 103.2999) (26.5003, 103.3037) (26.5084, 103.3074) (26.5164, 103.3113) (26.5244, 103.3153) (26.5323, 103.3193) (26.5402, 103.3233) (26.548, 103.3275) (26.5559, 103.3317) (26.5637, 103.3361) (26.5715, 103.3405) (26.5793, 103.3449) (26.5871, 103.3495) (26.5948, 103.3541) (26.6026, 103.3588) (26.6104, 103.3636) (26.6181, 103.3684) (26.626, 103.3733) (26.6337, 103.3784) (26.6415, 103.3835) (26.6494, 103.3886) (26.6572, 103.3939) (26.665, 103.3992) (26.6729, 103.4047) (26.6808, 103.4102) (26.6887, 103.4158) (26.6967, 103.4215) (26.7047, 103.4273) (26.7126, 103.4331) (26.7207, 103.4391) (26.7287, 103.4452) (26.7367, 103.4512) (26.7727, 103.4783) (26.8088, 103.5051) (26.8453, 103.5314) (26.873, 103.5512) (26.9008, 103.5708) (26.9288, 103.5902) (26.96, 103.6118) (26.9914, 103.633) (27.023, 103.6541) (27.0578, 103.6772) (27.0929, 103.7001) (27.1281, 103.7226) (27.1666, 103.7473) (27.2053, 103.7716) (27.2442, 103.7955) (27.2865, 103.8215) (27.3289, 103.8471) (27.3716, 103.8723) (27.4177, 103.8995) (27.4639, 103.9263) (27.5105, 103.9527) (27.5603, 103.981) (27.6105, 104.0089) (27.6609, 104.0363) (27.7147, 104.0656) (27.7688, 104.0944) (27.8231, 104.1227) (27.8808, 104.1528) (27.9389, 104.1824) (27.9972, 104.2114) (28.0589, 104.2423) (28.121, 104.2725) (28.1833, 104.3022) (28.2491, 104.3336) (28.3152, 104.3644) (28.3815, 104.3946) (28.5043, 104.4505) (28.6279, 104.5044) (28.7523, 104.5565) knots 0 0 0 0 0.057795 0.057795 0.057795 0.089038 0.089038 0.089038 0.118617 0.118617 0.118617 0.14653 0.14653 0.14653 0.172778 0.172778 0.172778 0.19736 0.19736 0.19736 0.220277 0.220277 0.220277 0.241529 0.241529 0.241529 0.261115 0.261115 0.261115 0.279036 0.279036 0.279036 0.295292 0.295292 0.295292 0.309882 0.309882 0.309882 0.329164 0.329164 0.329164 0.333477 0.333477 0.333477 0.337694 0.337694 0.337694 0.34182 0.34182 0.34182 0.345864 0.345864 0.345864 0.349834 0.349834 0.349834 0.353742 0.353742 0.353742 0.3576 0.3576 0.3576 0.361424 0.361424 0.361424 0.365232 0.365232 0.365232 0.369048 0.369048 0.369048 0.372899 0.372899 0.372899 0.376819 0.376819 0.376819 0.380853 0.380853 0.380853 0.385052 0.385052 0.385052 0.389482 0.389482 0.389482 0.394225 0.394225 0.394225 0.399381 0.399381 0.399381 0.405067 0.405067 0.405067 0.411413 0.411413 0.411413 0.418548 0.418548 0.418548 0.426565 0.426565 0.426565 0.435472 0.435472 0.435472 0.445133 0.445133 0.445133 0.45436 0.45436 0.45436 0.5 0.5 0.5 0.54564 0.54564 0.54564 0.554867 0.554867 0.554867 0.564528 0.564528 0.564528 0.573435 0.573435 0.573435 0.581452 0.581452 0.581452 0.588587 0.588587 0.588587 0.594933 0.594933 0.594933 0.600619 0.600619 0.600619 0.605775 0.605775 0.605775 0.610518 0.610518 0.610518 0.614948 0.614948 0.614948 0.619147 0.619147 0.619147 0.623181 0.623181 0.623181 0.627101 0.627101 0.627101 0.630952 0.630952 0.630952 0.634768 0.634768 0.634768 0.638576 0.638576 0.638576 0.6424 0.6424 0.6424 0.646258 0.646258 0.646258 0.650166 0.650166 0.650166 0.654136 0.654136 0.654136 0.65818 0.65818 0.65818 0.662306 0.662306 0.662306 0.666523 0.666523 0.666523 0.670836 0.670836 0.670836 0.690118 0.690118 0.690118 0.704708 0.704708 0.704708 0.720964 0.720964 0.720964 0.738885 0.738885 0.738885 0.758471 0.758471 0.758471 0.779723 0.779723 0.779723 0.80264 0.80264 0.80264 0.827222 0.827222 0.827222 0.85347 0.85347 0.85347 0.881383 0.881383 0.881383 0.910962 0.910962 0.910962 0.942205 0.942205 0.942205 1 1 1 1
  arc A204 (26.6454, 106.6388) -> (25.779, 107.4098) centre (0.0435, 77.6158) ccw
  spline S3 degree 3 poles (23.466, 109.2604) (23.4287, 109.1308) (23.3895, 109.0018) (23.3483, 108.8734) (23.326, 108.8039) (23.3031, 108.7347) (23.2795, 108.6657) (23.2573, 108.6004) (23.2344, 108.5352) (23.211, 108.4703) (23.1889, 108.409) (23.1663, 108.348) (23.1431, 108.2871) (23.1213, 108.2299) (23.099, 108.1728) (23.0761, 108.116) (23.0548, 108.0627) (23.0329, 108.0097) (23.0106, 107.9569) (22.9898, 107.9076) (22.9686, 107.8585) (22.9469, 107.8096) (22.9268, 107.7643) (22.9063, 107.7191) (22.8854, 107.6742) (22.8661, 107.6327) (22.8465, 107.5914) (22.8265, 107.5503) (22.8082, 107.5127) (22.7896, 107.4753) (22.7706, 107.438) (22.7534, 107.4042) (22.7359, 107.3705) (22.7181, 107.337) (22.7021, 107.307) (22.6859, 107.277) (22.6694, 107.2473) (22.6475, 107.2079) (22.6251, 107.1689) (22.6024, 107.1301) (22.5973, 107.1214) (22.5922, 107.1127) (22.5872, 107.104) (22.5823, 107.0955) (22.5775, 107.0869) (22.5728, 107.0782) (22.5681, 107.0698) (22.5636, 107.0613) (22.5591, 107.0528) (22.5547, 107.0445) (22.5504, 107.0361) (22.5461, 107.0276) (22.542, 107.0193) (22.5379, 107.011) (22.5339, 107.0027) (22.53, 106.9944) (22.5262, 106.9862) (22.5224, 106.9779) (22.5187, 106.9696) (22.5151, 106.9614) (22.5116, 106.9531) (22.5081, 106.9449) (22.5047, 106.9366) (22.5015, 106.9283) (22.4982, 106.9201) (22.4951, 106.9117) (22.492, 106.9034) (22.489, 106.895) (22.4861, 106.8866) (22.4833, 106.8781) (22.4805, 106.8696) (22.4779, 106.861) (22.4753, 106.8524) (22.4728, 106.8436) (22.4704, 106.8348) (22.4681, 106.8259) (22.4658, 106.8168) (22.4637, 106.8076) (22.4618, 106.7984) (22.4598, 106.7888) (22.458, 106.7792) (22.4565, 106.7695) (22.4548, 106.7593) (22.4535, 106.749) (22.4524, 106.7387) (22.4512, 106.7277) (22.4503, 106.7167) (22.4498, 106.7056) (22.4493, 106.6936) (22.4492, 106.6816) (22.4495, 106.6695) (22.4498, 106.6563) (22.4507, 106.643) (22.4521, 106.6298) (22.4536, 106.6151) (22.4559, 106.6004) (22.4589, 106.5859) (22.4622, 106.5696) (22.4665, 106.5535) (22.4716, 106.5376) (22.4774, 106.5198) (22.4843, 106.5024) (22.4923, 106.4854) (22.5012, 106.4667) (22.5115, 106.4485) (22.523, 106.4312) (22.5356, 106.4124) (22.5496, 106.3946) (22.565, 106.3782) (22.5798, 106.3625) (22.5959, 106.3482) (22.6122, 106.3341) (22.6931, 106.2645) (22.7794, 106.2021) (22.8626, 106.1356) (22.9457, 106.0691) (23.0256, 105.9985) (23.1112, 105.9349) (23.1285, 105.922) (23.146, 105.9094) (23.1645, 105.8985) (23.1839, 105.887) (23.2044, 105.8773) (23.2255, 105.8692) (23.2449, 105.8617) (23.2649, 105.8556) (23.2852, 105.8511) (23.3034, 105.8469) (23.322, 105.844) (23.3406, 105.8423) (23.3572, 105.8408) (23.3739, 105.8402) (23.3905, 105.8405) (23.4053, 105.8408) (23.4201, 105.8418) (23.4348, 105.8435) (23.448, 105.845) (23.4611, 105.8471) (23.4742, 105.8497) (23.486, 105.852) (23.4977, 105.8548) (23.5093, 105.8579) (23.52, 105.8609) (23.5306, 105.8641) (23.541, 105.8677) (23.5508, 105.871) (23.5605, 105.8746) (23.5701, 105.8784) (23.5792, 105.8821) (23.5882, 105.8859) (23.5972, 105.89) (23.6057, 105.8939) (23.6142, 105.8979) (23.6226, 105.9022) (23.6308, 105.9063) (23.6389, 105.9106) (23.6469, 105.915) (23.6547, 105.9194) (23.6625, 105.9239) (23.6703, 105.9285) (23.6779, 105.933) (23.6855, 105.9377) (23.693, 105.9425) (23.7005, 105.9473) (23.7079, 105.9522) (23.7152, 105.9572) (23.7226, 105.9622) (23.7299, 105.9673) (23.7372, 105.9725) (23.7445, 105.9777) (23.7518, 105.983) (23.759, 105.9885) (23.7663, 105.9939) (23.7735, 105.9995) (23.7807, 106.0051) (23.7879, 106.0109) (23.7952, 106.0167) (23.8023, 106.0225) (23.8096, 106.0285) (23.8169, 106.0346) (23.824, 106.0407) (23.8314, 106.0469) (23.8386, 106.0533) (23.8459, 106.0596) (23.8532, 106.0661) (23.8606, 106.0727) (23.8678, 106.0793) (23.8752, 106.0861) (23.8826, 106.093) (23.89, 106.0999) (23.9229, 106.1306) (23.956, 106.161) (23.9896, 106.191) (24.015, 106.2136) (24.0407, 106.236) (24.0665, 106.2582) (24.0953, 106.2829) (24.1243, 106.3073) (24.1535, 106.3316) (24.1857, 106.3582) (24.2181, 106.3846) (24.2508, 106.4107) (24.2865, 106.4393) (24.3225, 106.4675) (24.3587, 106.4953) (24.398, 106.5256) (24.4375, 106.5555) (24.4774, 106.5851) (24.5203, 106.6169) (24.5635, 106.6484) (24.607, 106.6795) (24.6537, 106.7129) (24.7007, 106.7458) (24.7479, 106.7784) (24.7983, 106.8131) (24.8491, 106.8474) (24.9002, 106.8812) (24.9545, 106.9172) (25.0091, 106.9527) (25.064, 106.9877) (25.1222, 107.0248) (25.1808, 107.0614) (25.2396, 107.0974) (25.3018, 107.1355) (25.3643, 107.173) (25.4271, 107.21) (25.5434, 107.2784) (25.6607, 107.345) (25.779, 107.4098) knots 0 0 0 0 0.057795 0.057795 0.057795 0.089038 0.089038 0.089038 0.118617 0.118617 0.118617 0.14653 0.14653 0.14653 0.172778 0.172778 0.172778 0.19736 0.19736 0.19736 0.220277 0.220277 0.220277 0.241529 0.241529 0.241529 0.261115 0.261115 0.261115 0.279036 0.279036 0.279036 0.295292 0.295292 0.295292 0.309882 0.309882 0.309882 0.329164 0.329164 0.329164 0.333477 0.333477 0.333477 0.337694 0.337694 0.337694 0.34182 0.34182 0.34182 0.345864 0.345864 0.345864 0.349834 0.349834 0.349834 0.353742 0.353742 0.353742 0.3576 0.3576 0.3576 0.361424 0.361424 0.361424 0.365232 0.365232 0.365232 0.369048 0.369048 0.369048 0.372899 0.372899 0.372899 0.376819 0.376819 0.376819 0.380853 0.380853 0.380853 0.385052 0.385052 0.385052 0.389482 0.389482 0.389482 0.394225 0.394225 0.394225 0.399381 0.399381 0.399381 0.405067 0.405067 0.405067 0.411413 0.411413 0.411413 0.418548 0.418548 0.418548 0.426565 0.426565 0.426565 0.435472 0.435472 0.435472 0.445133 0.445133 0.445133 0.45436 0.45436 0.45436 0.5 0.5 0.5 0.54564 0.54564 0.54564 0.554867 0.554867 0.554867 0.564528 0.564528 0.564528 0.573435 0.573435 0.573435 0.581452 0.581452 0.581452 0.588587 0.588587 0.588587 0.594933 0.594933 0.594933 0.600619 0.600619 0.600619 0.605775 0.605775 0.605775 0.610518 0.610518 0.610518 0.614948 0.614948 0.614948 0.619147 0.619147 0.619147 0.623181 0.623181 0.623181 0.627101 0.627101 0.627101 0.630952 0.630952 0.630952 0.634768 0.634768 0.634768 0.638576 0.638576 0.638576 0.6424 0.6424 0.6424 0.646258 0.646258 0.646258 0.650166 0.650166 0.650166 0.654136 0.654136 0.654136 0.65818 0.65818 0.65818 0.662306 0.662306 0.662306 0.666523 0.666523 0.666523 0.670836 0.670836 0.670836 0.690118 0.690118 0.690118 0.704708 0.704708 0.704708 0.720964 0.720964 0.720964 0.738885 0.738885 0.738885 0.758471 0.758471 0.758471 0.779723 0.779723 0.779723 0.80264 0.80264 0.80264 0.827222 0.827222 0.827222 0.85347 0.85347 0.85347 0.881383 0.881383 0.881383 0.910962 0.910962 0.910962 0.942205 0.942205 0.942205 1 1 1 1
  arc A205 (23.466, 109.2604) -> (22.5237, 109.9366) centre (0.0435, 77.6158) ccw